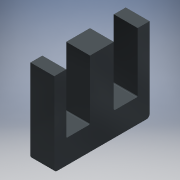
# Autodesk Inventor part: coil 55_28_21-02
Saved by Autodesk Inventor 2019 (Build 230136000, 136)
## iProperties
Created: 2017-05-26
Part Number: coil 55_28_21-02
Material: Generic
Document SubType Name: Modeling
Designer: ppapaman
Density: 1 g/cm^3
Appearance: Iron Gray
Mass: 138.558 g
Surface Area: 270.616 cm^2
Volume: 138.558 cm^3
Author: ppapaman
Autodesk Inventor part; units mm, degrees
ref_plane "YZ Plane" through (0, 0, 0) normal (1, 0, 0) x (0, 1, 0)
ref_plane "XZ Plane" through (0, 0, 0) normal (0, 1, 0) x (-1, 0, 0)
ref_plane "XY Plane" through (0, 0, 0) normal (0, 0, 1) x (1, 0, 0)
sketch "Sketch1" plane through (0, 0, 0) normal (0, 1, 0) x (-1, 0, 0)
  line L0 (10, 40) -> (-10, 40)
  line L1 (-10, 40) -> (-10, -40)
  line L2 (-10, -40) -> (10, -40)
  line L3 (10, -40) -> (10, 40)
  point P0 (0, 0)
  point P1 (10, 0)
  point P2 (0, -40)
  dimension "d0" = 80
  dimension "d1" = 20
  constraints: 8 end point, 2 midpoint, 2 parallel, 1 horizontal, 1 horizontal alignment, 1 perpendicular, 1 vertical alignment
  measures "d0" distance between parallel lines of L2 L0
  measures "d1" distance between parallel lines of L1 L3
extrude "MainCore" add sketch "Sketch1" along normal blind 70
sketch "Sketch3" plane through (0, 70, 0) normal (0, 1, 0) x (1, 0, 0)
  line L0 (-10, -10) -> (10, -10)
  line L1 (10, -10) -> (10, 10)
  line L2 (10, 10) -> (-10, 10)
  line L3 (-10, 10) -> (-10, -10)
  line L4 (-10, 40) -> (-10, -40) projected
  line L5 (-10, -30) -> (10, -30)
  line L6 (10, -30) -> (10, -10)
  line L7 (10, -10) -> (-10, -10)
  line L8 (-10, -10) -> (-10, -30)
  line L9 (-10, 10) -> (10, 10)
  line L10 (10, 10) -> (10, 30)
  line L11 (10, 30) -> (-10, 30)
  line L12 (-10, 30) -> (-10, 10)
  point P0 (0, 0)
  point P1 (-10, 0)
  point P2 (0, 10)
  point P3 (0, -10)
  point P4 (0, 10)
  dimension "d4" = 20
  dimension "d5" = 20
  dimension "d6" = 20
  constraints: 24 end point, 6 parallel, 5 collinear, 4 midpoint, 3 horizontal, 3 perpendicular, 3 vertical alignment, 1 horizontal alignment
  measures "d4" distance between parallel lines of L2 L0
  measures "d5" distance between parallel lines of L0 L5
  measures "d6" distance between parallel lines of L11 L2
extrude "Windows" cut sketch "Sketch3" against normal blind 50 contours L0 L6 L5 L4 | L4 L11 L10 L2
fillet "Outer corners" radius 2.4 2 edges at (0, 0, -40) (0, 0, 40)
fillet "Fillet2" radius 1 4 edges at (0, 20, 10) (0, 20, 30) (0, 20, -10) (0, 20, -30)
equation "\"d0\" = coreWidth"
equation "\"d1\" = coreDepth"
equation "\"d4\" = coreLegWidthInner"
equation "\"d5\" = -0.5 * coreLegWidthInner + 0.5 * coreWidthInner"
equation "\"d6\" = -0.5 * coreLegWidthInner + 0.5 * coreWidthInner"
equation "\"d9\" = 0.03 * coreWidth"
equation "\"d10\" = 0.025 * coreWidthInner - 0.025 * coreLegWidthInner"
equation "\"coreWidth\" = 80"
equation "\"coreDepth\" = 20"
equation "\"coreLegWidthInner\" = 20"
equation "\"wallThick\" = 1"
equation "\"extDepth\" = 271.8"
equation "\"WireDia\" = 1.2"
equation "\"Airgap\" = 0.24"
equation "\"coreWidthInner\" = 60"
body "Solid1"
